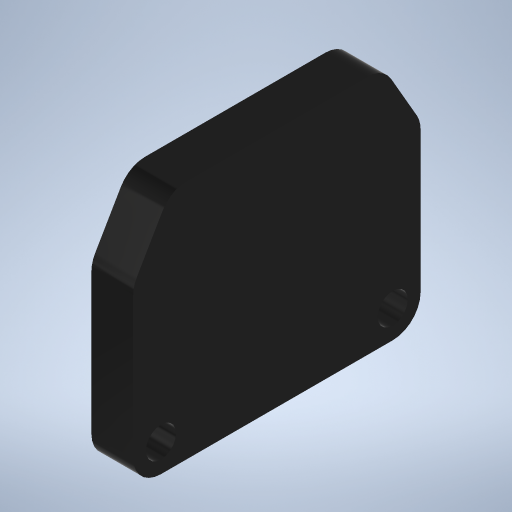
# Autodesk Inventor part: Tool_Template
Saved by Autodesk Inventor 2023.2 (Build 272271000, 271)
## iProperties
Created: 2022-06-19
Part Number: Tool_Template
Material: ABS Plastic
Document SubType Name: Modeling
Designer: Remo
Density: 1.06 g/cm^3
Appearance: Smooth - Black
Author: Remo
Autodesk Inventor part; units mm, degrees
ref_plane "YZ Plane" through (0, 0, 0) normal (1, 0, 0) x (0, 1, 0)
ref_plane "XZ Plane" through (0, 0, 0) normal (0, 1, 0) x (-1, 0, 0)
ref_plane "XY Plane" through (0, 0, 0) normal (0, 0, 1) x (1, 0, 0)
sketch "Sketch1" plane through (0, 0, 0) normal (1, 0, 0) x (0, 1, 0)
  circle A0 centre (8.9201, -5.15) radius 5.15
  circle A1 centre (8.9201, 5.15) radius 5.15
  circle A2 centre (0, 10.3) radius 5.15
  circle A3 centre (-8.9201, 5.15) radius 5.15
  circle A4 centre (-8.9201, -5.15) radius 5.15
  circle A5 centre (0, -10.3) radius 5.15
  line L0 (-27.5, 7.5) -> (-16.5, 7.5)
  line L1 (-16.5, 7.5) -> (-16.5, -7.5)
  line L2 (-16.5, -7.5) -> (-27.5, -7.5)
  line L3 (-27.5, -7.5) -> (-27.5, 7.5)
  line L4 (-27.5, 7.5) -> (-16.5, -7.5) construction
  line L5 (-16.5, 7.5) -> (-27.5, -7.5) construction
  line L6 (14.7452, -10.5394) -> (20.2452, -20.0657)
  line L7 (1.7548, -18.0394) -> (14.7452, -10.5394)
  line L8 (7.2548, -27.5657) -> (1.7548, -18.0394)
  line L9 (20.2452, -20.0657) -> (7.2548, -27.5657)
  line L10 (1.7548, 18.0394) -> (7.2548, 27.5657)
  line L11 (14.7452, 10.5394) -> (1.7548, 18.0394)
  line L12 (20.2452, 20.0657) -> (14.7452, 10.5394)
  line L13 (7.2548, 27.5657) -> (20.2452, 20.0657)
  circle A6 centre (-22, 25) radius 3.25
  circle A7 centre (-22, -25) radius 3.25
  arc A8 (-22, 31) -> (-28, 25) centre (-22, 25) ccw
  arc A9 (-28, -25) -> (-22, -31) centre (-22, -25) ccw
  line L14 (-28, 25) -> (-28, -25)
  line L15 (-22, 31) -> (10, 31)
  line L16 (10, -31) -> (-22, -31)
  line L17 (10, -31) -> (24, -22.9171)
  line L18 (24, -22.9171) -> (24, 22.9171)
  line L19 (24, 22.9171) -> (10, 31)
  point P0 (0, 0)
  point P1 (-22, 0)
  point P2 (-4.46, -7.725)
  point P3 (-8.9201, 0)
  point P4 (-4.46, 7.725)
  point P5 (4.46, 7.725)
  point P6 (8.9201, 0)
  point P7 (4.46, -7.725)
  dimension "d0" = 10.3
  dimension "d3" = 360
  dimension "d5" = 15
  dimension "d6" = 11
  dimension "d7" = 22
  dimension "d10" = 360
  dimension "d12" = 25
  dimension "d13" = 50
  dimension "d14" = 6.5
  dimension "d15" = 12
  dimension "d29" = 10
  dimension "d31" = 24
  constraints: 40 end point, 10 centre point, 4 parallel, 4 point on circle, 4 tangent, 4 vertical alignment, 3 horizontal, 2 coincident, 2 equal radius, 2 midpoint, 2 vertical, 1 horizontal alignment, 1 perpendicular, 38 other
  measures "d0" diameter of A0
  measures "d5" distance of L2.end L0.start
  measures "d6" distance of L1.end L2.end
  measures "d7" distance of point (-22, 0) point (0, 0)
  measures "d12" vertical distance of point (0, 0) A6.centre
  measures "d13" distance of A6.centre A7.centre
  measures "d14" diameter of A6
  measures "d15" diameter of A8
  measures "d29" horizontal distance of L16.start point (0, 0)
  measures "d31" distance from line of point (0, 0) L18
extrude "Layer1_Magnets_16" add sketch "Sketch1" along normal blind 1.6 contours A0 A5 A4 A3 A2 A1 | L15 L19 L18 L17 L16 A9 L14 A8
sketch "Sketch2" plane through (1.6, 0, 0) normal (1, 0, 0) x (0, 0, -1)
  arc A0 (-31, -22) -> (-25, -28) centre (-25, -22) ccw projected
  line L0 (-25, -28) -> (25, -28) projected
  arc A1 (25, -28) -> (31, -22) centre (25, -22) ccw projected
  line L1 (31, -22) -> (31, 10) projected
  line L2 (-31, 10) -> (-31, -22) projected
  arc A2 (7.725, -4.46) -> (7.725, 4.46) centre (10.3, 0) ccw projected
  arc A3 (0, -8.9201) -> (7.725, -4.46) centre (5.15, -8.9201) ccw projected
  arc A4 (-7.725, -4.46) -> (0, -8.9201) centre (-5.15, -8.9201) ccw projected
  arc A5 (-7.725, 4.46) -> (-7.725, -4.46) centre (-10.3, 0) ccw projected
  arc A6 (0, 8.9201) -> (-7.725, 4.46) centre (-5.15, 8.9201) ccw projected
  arc A7 (7.725, 4.46) -> (0, 8.9201) centre (5.15, 8.9201) ccw projected
  circle A8 centre (25, -22) radius 3.25 projected
  circle A9 centre (-25, -22) radius 3.25 projected
  line L3 (-18.0394, 1.7548) -> (-27.5657, 7.2548) projected
  line L4 (-27.5657, 7.2548) -> (-20.0657, 20.2452) projected
  line L5 (-20.0657, 20.2452) -> (-10.5394, 14.7452) projected
  line L6 (-10.5394, 14.7452) -> (-18.0394, 1.7548) projected
  line L7 (10.5394, 14.7452) -> (20.0657, 20.2452) projected
  line L8 (20.0657, 20.2452) -> (27.5657, 7.2548) projected
  line L9 (27.5657, 7.2548) -> (18.0394, 1.7548) projected
  line L10 (18.0394, 1.7548) -> (10.5394, 14.7452) projected
  line L11 (-7.5, -27.5) -> (-7.5, -16.5) projected
  line L12 (-7.5, -16.5) -> (7.5, -16.5) projected
  line L13 (7.5, -16.5) -> (7.5, -27.5) projected
  line L14 (7.5, -27.5) -> (-7.5, -27.5) projected
  arc A10 (0, 8.9201) -> (7.725, 4.46) centre (5.15, 8.9201) ccw projected
  arc A11 (-7.725, 4.46) -> (0, 8.9201) centre (-5.15, 8.9201) ccw projected
  arc A12 (-7.725, -4.46) -> (-7.725, 4.46) centre (-10.3, 0) ccw projected
  arc A13 (0, -8.9201) -> (-7.725, -4.46) centre (-5.15, -8.9201) ccw projected
  arc A14 (7.725, -4.46) -> (0, -8.9201) centre (5.15, -8.9201) ccw projected
  arc A15 (7.725, 4.46) -> (7.725, -4.46) centre (10.3, 0) ccw projected
  line L15 (31, 10) -> (22.9171, 24) projected
  line L16 (22.9171, 24) -> (-22.9171, 24) projected
  line L17 (-22.9171, 24) -> (-31, 10) projected
  point P0 (0, 0)
  point P1 (-7.725, 4.46)
  point P2 (-7.725, 4.46)
  point P3 (-7.725, 4.46)
  point P4 (-7.725, -4.46)
  point P5 (-7.725, -4.46)
  point P6 (-7.725, -4.46)
  point P7 (-7.725, -4.46)
  point P8 (0, -8.9201)
  point P9 (0, -8.9201)
  point P10 (0, -8.9201)
  point P11 (7.725, 4.46)
  point P12 (7.725, 4.46)
  point P13 (0, 8.9201)
  point P14 (0, 8.9201)
extrude "Layer2_Coupler_80" add sketch "Sketch2" along normal blind 6.4 contours L2 L17 L16 L15 L1 A1 L0 A0 | A15 A2 | A3 A14 | A14 A13 A12 A11 A10 A15 | A10 A7 | A4 A13 | A11 A6 | A5 A12
sketch "Sketch3" plane through (8, 0, 0) normal (1, 0, 0) x (0, 0, -1)
  circle A0 centre (25, -22) radius 3.25 projected
  circle A1 centre (-25, -22) radius 3.25 projected
  line L0 (-18.0394, 1.7548) -> (-27.5657, 7.2548) projected
  line L1 (-27.5657, 7.2548) -> (-20.0657, 20.2452) projected
  line L2 (-20.0657, 20.2452) -> (-10.5394, 14.7452) projected
  line L3 (-10.5394, 14.7452) -> (-18.0394, 1.7548) projected
  line L4 (10.5394, 14.7452) -> (20.0657, 20.2452) projected
  line L5 (20.0657, 20.2452) -> (27.5657, 7.2548) projected
  line L6 (27.5657, 7.2548) -> (18.0394, 1.7548) projected
  line L7 (18.0394, 1.7548) -> (10.5394, 14.7452) projected
  line L8 (-7.5, -27.5) -> (-7.5, -16.5) projected
  line L9 (-7.5, -16.5) -> (7.5, -16.5) projected
  line L10 (7.5, -16.5) -> (7.5, -27.5) projected
  line L11 (7.5, -27.5) -> (-7.5, -27.5) projected
  line L12 (-25, -28) -> (25, -28) projected
  arc A2 (25, -28) -> (31, -22) centre (25, -22) ccw projected
  line L13 (31, -22) -> (31, 10) projected
  line L14 (-31, 10) -> (-31, -22) projected
  arc A3 (-31, -22) -> (-25, -28) centre (-25, -22) ccw projected
  line L15 (22.9171, 24) -> (-22.9171, 24) projected
  line L16 (-22.9171, 24) -> (-31, 10) projected
  line L17 (31, 10) -> (22.9171, 24) projected
  point P0 (0, 0)
extrude "Layer3_Cover_90" add sketch "Sketch3" along normal blind 1 contours L0 L1 L2 L3 | L4 L5 L6 L7 | L8 L9 L10 L11 | A3 L14 L16 L15 L17 L13 A2 L12
chamfer "CouplerL" distance 7.5 angle 45 6 edges at (8, -22, 7.5) (8, -22, -7.5) (8, 4.5048, -22.8026) (8, 17.4952, -15.3026) (8, 17.4952, 15.3026) (8, 4.5048, 22.8026)
fillet "EdgeRadius" radius 6 4 edges at (4.5, 10, -31) (4.5, 10, 31) (4.5, 24, 22.9171) (4.5, 24, -22.9171)
equation "\"d13\" = 2 * d12"
body "Solid1"
